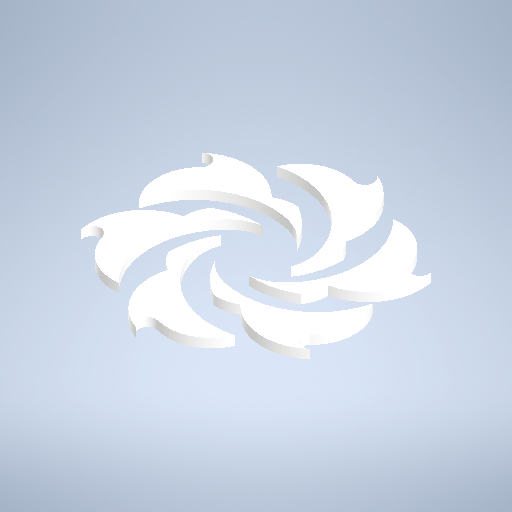
# Autodesk Inventor part: LOGO
Saved by Autodesk Inventor 2026.1 (Build 301233020, 233B)
## iProperties
Created: 2025-07-18
Part Number: LOGO
Material: 一般
Document SubType Name: Modeling
Designer: hibik
Density: 1 g/cm^3
Appearance: 既定
Author: hibik
Autodesk Inventor part; units mm, degrees
ref_plane "YZ Plane" through (0, 0, 0) normal (1, 0, 0) x (0, 1, 0)
ref_plane "XZ Plane" through (0, 0, 0) normal (0, 1, 0) x (-1, 0, 0)
ref_plane "XY Plane" through (0, 0, 0) normal (0, 0, 1) x (1, 0, 0)
sketch "スケッチ1" plane through (0, 0, 0) normal (0, 1, 0) x (-1, 0, 0)
  circle A0 centre (0, 0) radius 150 construction
  arc A1 (-37.6897, 7.8571) -> (29.3443, -24.9231) centre (0, 0) ccw
  arc A2 (-37.6897, 7.8571) -> (87.1485, -88.2381) centre (47.9687, -10) ccw
  arc A3 (29.3443, -24.9231) -> (87.1485, -88.2381) centre (26.6834, -85.3964) ccw
  arc A4 (12.5, -123.4123) -> (6.6984, -142.534) centre (10, -133.0948) ccw
  arc A5 (29.1319, -25.171) -> (71.0869, -94.3908) centre (25, -75) ccw
  arc A6 (-48.3693, -50) -> (-39.4956, -7.5004) centre (-14, -35) ccw
  arc A7 (-35, -4) -> (-35.786, -35.3257) centre (12.0738, -20.8539) ccw
  arc A8 (-35, -4) -> (-48.3693, -50) centre (36.6303, -49.7613) ccw
  point P0 (-31.3653, -68.237)
  point P1 (6.6984, -142.534)
  point P2 (12.5, -123.4123)
  point P3 (71.0869, -94.3908)
  point P4 (-13.2756, -72.493)
  point P5 (-24.8317, -70.9016)
  point P6 (-23.0378, -61.1304)
  point P7 (-39.4956, -7.5004)
  point P8 (87.1485, -88.2381)
  point P9 (22.1516, -25.0345)
  point P10 (-26.341, -56.1986)
  point P11 (17.008, -25.6428)
  point P12 (22.1643, -25.0805)
  point P13 (23.251, -30.6861)
  point P14 (63.4693, -48.0608)
  point P15 (-36.9251, -10.8989)
  point P16 (-37.5882, -8.3293)
  point P17 (-39.509, -11.975)
  point P18 (-36.7334, -7.086)
  point P19 (-37.6897, 7.8571)
  point P20 (-35.7696, -6.328)
  point P21 (-37.9998, -6.1858)
  dimension "d0" = 300
  dimension "d1" = 77
  dimension "d7" = 20
  dimension "d9" = 25
  dimension "d10" = 75
  dimension "d11" = 100
  dimension "d13" = 75
  dimension "d15" = 35
  dimension "d16" = 14
  dimension "d17" = 10
  dimension "d18" = 10
  dimension "d19" = 175
  dimension "d20" = 35
  dimension "d21" = 4
  dimension "d23" = 15
  dimension "d24" = 85
  dimension "d25" = 50
  constraints: 22 point on circle, 9 centre point, 6 tangent, 2 coincident
  measures "d0" diameter of A0
  measures "d1" diameter of A1
  measures "d7" diameter of A4
  measures "d9" horizontal distance of point (0, 0) A5.centre
  measures "d10" vertical distance of point (0, 0) A5.centre
  measures "d11" diameter of A5
  measures "d13" diameter of A6
  measures "d15" vertical distance of point (0, 0) A6.centre
  measures "d16" horizontal distance of point (0, 0) A6.centre
  measures "d17" vertical distance of point (0, 0) A2.centre
  measures "d18" horizontal distance of point (0, 0) A4.centre
  measures "d19" diameter of A2
  measures "d20" horizontal distance of point (0, 0) A7.start
  measures "d21" vertical distance of A7.start point (0, 0)
  measures "d23" vertical distance of A6.centre A6.start
  measures "d24" radius of A8
  measures "d25" radius of A7
extrude "押し出し1" add sketch "スケッチ1" along normal blind 10 contours A6 A5 A2 | A2 A5 A6 | A5 A6 A3 A2 | A5 A4 A3 A6 | A8 A7 A1 | A1 A7 A2 A8 | A3 A6 A8 A2
pattern_circular "円形状パターン1" count 6 over 360 about axis through (0, -10, 0) along (0, 1, 0) of "押し出し1"
sketch "スケッチ2" plane through (15.3241, 10, 46.5421) normal (0, 1, 0) x (0.999825, 0, -0.0187094)
  line L0 (-36.9278, 15.5633) -> (-52.759, 50.6578)
  line L1 (-52.759, 50.6578) -> (-30.2818, 81.9152)
  line L2 (-30.2818, 81.9152) -> (8.0265, 78.0781)
  line L3 (8.0265, 78.0781) -> (23.8577, 42.9836)
  line L4 (23.8577, 42.9836) -> (1.3805, 11.7262)
  line L5 (1.3805, 11.7262) -> (-36.9278, 15.5633)
  circle A0 centre (-14.4507, 46.8207) radius 38.5
  point P0 (-29.0886, 14.7781)
  point P1 (-49.5194, 43.4762)
  point P2 (-34.8814, 75.5189)
  point P3 (0.1873, 78.8633)
  point P4 (20.6181, 50.1652)
  point P5 (5.9801, 18.1225)
  dimension "d27" = 77
  constraints: 12 end point, 2 coincident, 1 point on line, 16 other
ref_plane "作業平面1" through (16.485, 10, 34.7922) normal (0.0810308, 0, -0.9967116) x (-0.9967116, 0, -0.0810308)
